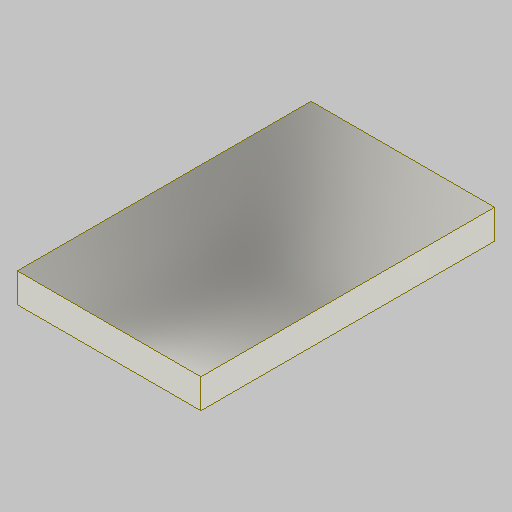
# Autodesk Inventor part: Part1
Saved by Autodesk Inventor 2025.2 (Build 292293000, 293)
## iProperties
Created: 2025-04-10
Part Number: Part1
Material: Silver
Document SubType Name: Modeling
Designer: joaki
Density: 10.49 g/cm^3
Appearance: Silver
Mass: 41.96 g
Surface Area: 25.2 cm^2
Volume: 4 cm^3
Author: joaki
Autodesk Inventor part; units mm, degrees
ref_plane "YZ Plane" through (0, 0, 0) normal (1, 0, 0) x (0, 1, 0)
ref_plane "XZ Plane" through (0, 0, 0) normal (0, 1, 0) x (-1, 0, 0)
ref_plane "XY Plane" through (0, 0, 0) normal (0, 0, 1) x (1, 0, 0)
sketch "Sketch1" plane through (0, 0, 0) normal (0, 1, 0) x (-1, 0, 0)
  line L0 (26.533, 42.9481) -> (1.533, 42.9481)
  line L1 (1.533, 42.9481) -> (1.533, 2.9481)
  line L2 (1.533, 2.9481) -> (26.533, 2.9481)
  line L3 (26.533, 2.9481) -> (26.533, 42.9481)
  point P0 (0, 0)
  dimension "d0" = 25
  dimension "d1" = 40
  constraints: 8 end point, 2 parallel, 1 horizontal, 1 perpendicular
  measures "d0" distance between parallel lines of L3 L1
  measures "d1" distance between parallel lines of L2 L0
extrude "Extrusion1" add sketch "Sketch1" along normal blind 4
body "Solid1"
